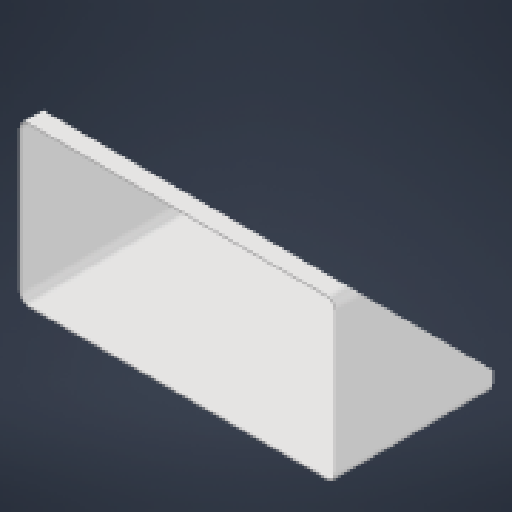
# Autodesk Inventor part: Body Cover
Saved by Autodesk Inventor 2023 (Build 270158000, 158)
## iProperties
Created: 2022-10-09
Part Number: Body Cover
Material: Aluminum 6061
Document SubType Name: Modeling
Designer: Hilal Yahya
Density: 2.7 g/cm^3
Appearance: Aluminum - Flat
Author: Hilal Yahya
Autodesk Inventor part; units mm, degrees
ref_plane "YZ Plane" through (0, 0, 0) normal (1, 0, 0) x (0, 1, 0)
ref_plane "XZ Plane" through (0, 0, 0) normal (0, 1, 0) x (-1, 0, 0)
ref_plane "XY Plane" through (0, 0, 0) normal (0, 0, 1) x (1, 0, 0)
sketch "Sketch1" plane through (0, 0, 0) normal (0, 0, 1) x (1, 0, 0)
  arc A0 (-140, 100) -> (-150, 90) centre (-140, 90) ccw projected
  line L0 (-140, 100) -> (140, 100) projected
  arc A1 (150, 90) -> (140, 100) centre (140, 90) ccw projected
  line L1 (150, 90) -> (150, -90) projected
  arc A2 (140, -100) -> (150, -90) centre (140, -90) ccw projected
  line L2 (140, -100) -> (-140, -100) projected
  arc A3 (-150, -90) -> (-140, -100) centre (-140, -90) ccw projected
  line L3 (-150, -90) -> (-150, 90) projected
  line L4 (-140, 100) -> (140, 100) projected
  arc A4 (-140, 100) -> (-150, 90) centre (-140, 90) ccw projected
  line L5 (-140, 100) -> (140, 100) projected
  arc A5 (150, 90) -> (140, 100) centre (140, 90) ccw projected
  line L6 (150, 90) -> (150, -90) projected
  arc A6 (140, -100) -> (150, -90) centre (140, -90) ccw projected
  line L7 (140, -100) -> (-140, -100) projected
  arc A7 (-150, -90) -> (-140, -100) centre (-140, -90) ccw projected
  line L8 (-150, -90) -> (-150, 90) projected
  line L9 (-190, 102) -> (190, 102)
  arc A8 (152, 90) -> (140, 102) centre (140, 90) ccw
  line L10 (152, 90) -> (152, -90)
  arc A9 (140, -102) -> (152, -90) centre (140, -90) ccw
  line L11 (190, -102) -> (-190, -102)
  arc A10 (-152, -90) -> (-140, -102) centre (-140, -90) ccw
  line L12 (-152, -90) -> (-152, 90)
  arc A11 (-140, 102) -> (-152, 90) centre (-140, 90) ccw
  point P0 (0, 0)
  point P1 (140, -102)
  point P2 (152, -90)
  point P3 (-140, 102)
  point P4 (-152, 90)
  dimension "d0" = 2
  dimension "d1" = 2
  dimension "d2" = 2
  dimension "d3" = 2
  dimension "d4" = 2
  dimension "d5" = 2
  dimension "d6" = 2
  dimension "d7" = 2
  constraints: 8 end point, 8 point on circle, 4 centre point, 4 parallel
  measures "d0" distance between parallel lines of L0 L9
  measures "d1" radial gap between concentric circles of A1 A8
  measures "d2" distance between parallel lines of L1 L10
  measures "d3" radial gap between concentric circles of A2 A9
  measures "d4" distance between parallel lines of L2 L11
  measures "d5" radial gap between concentric circles of A3 A10
  measures "d6" distance between parallel lines of L3 L12
  measures "d7" radial gap between concentric circles of A0 A11
extrude "Extrusion1" add sketch "Sketch1" against normal blind 200
sketch "Sketch2" plane through (152, -90, 0) normal (1, 0, 0) x (0, 0, -1)
  line L0 (0, 192) -> (200, 192) projected
  line L1 (0, -12) -> (200, -12) projected
  line L2 (0, 0) -> (0, 180) projected
  line L3 (200, 180) -> (200, 0) projected
  line L4 (0, 192) -> (200, 192) projected
  line L5 (23.2233, 192) -> (200, 15.2233)
  line L6 (200, 0) -> (200, 180) projected
  line L7 (23.2233, 192) -> (273.2233, 192) construction
  line L8 (200, 15.2233) -> (200, 192)
  point P0 (0, 90)
  point P1 (200, 180)
  point P2 (200, 15.2233)
  dimension "d10" = 45
  dimension "d11" = 250
  constraints: 6 end point, 2 point on line, 1 collinear, 1 equal length, 1 horizontal
  measures "d10" angle of L5 L7
  measures "d11" distance of L5.start L5.end
extrude "Extrusion2" cut sketch "Sketch2" against normal through all
body "Solid1"
